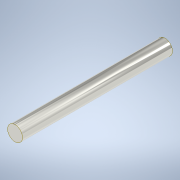
# Autodesk Inventor part: ステンレス平行ピンΦ3h7_30
Saved by Autodesk Inventor 2021 (Build 250183000, 183)
## iProperties
Created: 2021-10-20
Part Number: ステンレス平行ピンΦ3h7_30
Material: 一般
Document SubType Name: Modeling
Designer: ryusei
Density: 1 g/cm^3
Appearance: 銀
Author: ryusei
Autodesk Inventor part; units mm, degrees
ref_plane "YZ Plane" through (0, 0, 0) normal (1, 0, 0) x (0, 1, 0)
ref_plane "XZ Plane" through (0, 0, 0) normal (0, 1, 0) x (-1, 0, 0)
ref_plane "XY Plane" through (0, 0, 0) normal (0, 0, 1) x (1, 0, 0)
sketch "スケッチ1" plane through (0, 0, 0) normal (0, 0, 1) x (1, 0, 0)
  circle A0 centre (0, 0) radius 1.5
  dimension "d0" = 3
  constraints: 1 centre point, 1 coincident
  measures "d0" diameter of A0
extrude "押し出し1" add sketch "スケッチ1" along normal blind 30
